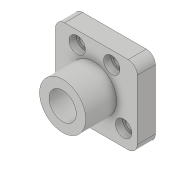
# Autodesk Inventor part: Mount_DMD_KM100
Saved by Autodesk Inventor 2019 (Build 230136000, 136)
## iProperties
Created: 2021-07-26
Part Number: Mount_DMD_KM100
Material: Generic
Document SubType Name: Modeling
Designer: wanghaoran
Density: 1 g/cm^3
Appearance: Default
Author: wanghaoran
Autodesk Inventor part; units mm, degrees
ref_plane "YZ Plane" through (0, 0, 0) normal (1, 0, 0) x (0, 1, 0)
ref_plane "XZ Plane" through (0, 0, 0) normal (0, 1, 0) x (-1, 0, 0)
ref_plane "XY Plane" through (0, 0, 0) normal (0, 0, 1) x (1, 0, 0)
sketch "Sketch1" plane through (0, 0, 0) normal (0, 0, 1) x (1, 0, 0)
  circle A0 centre (19, 0) radius 4.65 projected
  circle A1 centre (-6.5, -27) radius 4.65 projected
  circle A2 centre (0, 0) radius 4.65 projected
  circle A3 centre (25.5, -27) radius 4.65 projected
  arc A4 (28.02, -35.95) -> (33.02, -30.95) centre (28.02, -30.95) ccw projected
  line L0 (33.02, 2.05) -> (33.02, -30.95) projected
  arc A5 (33.02, 2.05) -> (28.02, 7.05) centre (28.02, 2.05) ccw projected
  line L1 (-6.98, 7.05) -> (28.02, 7.05) projected
  arc A6 (-6.98, 7.05) -> (-11.98, 2.05) centre (-6.98, 2.05) ccw projected
  line L2 (-11.98, -30.95) -> (-11.98, 2.05) projected
  arc A7 (-11.98, -30.95) -> (-6.98, -35.95) centre (-6.98, -30.95) ccw projected
  line L3 (28.02, -35.95) -> (-6.98, -35.95) projected
  arc A8 (20.169, -15.05) -> (19.169, -16.05) centre (20.169, -16.05) ccw projected
  line L4 (20.169, -15.05) -> (21.169, -15.05) projected
  line L5 (21.169, -15.05) -> (21.169, -17.95) projected
  line L6 (21.169, -17.95) -> (20.169, -17.95) projected
  arc A9 (19.169, -16.95) -> (20.169, -17.95) centre (20.169, -16.95) ccw projected
  line L7 (19.169, -16.95) -> (19.169, -22.1) projected
  line L8 (19.169, -22.1) -> (-2.331, -22.1) projected
  line L9 (-2.331, -22.1) -> (-2.331, -10.9) projected
  line L10 (-2.331, -10.9) -> (19.169, -10.9) projected
  line L11 (19.169, -10.9) -> (19.169, -16.05) projected
  circle A10 centre (-6.48, -12.9) radius 2 projected
  circle A11 centre (-3.844, -16.512) radius 0.75 projected
  circle A12 centre (23.72, -20.1) radius 2 projected
  line L12 (19.169, -16.05) -> (19.169, -16.95)
  circle A13 centre (25.5, -27) radius 3
  circle A14 centre (-6.5, -27) radius 3
  circle A15 centre (0, 0) radius 3
  circle A16 centre (19, 0) radius 3
  circle A17 centre (19, 0) radius 5
  dimension "d8" = 10
  dimension "d13" = 6
  dimension "d14" = 6
  dimension "d15" = 6
  dimension "d16" = 6
  constraints: 5 centre point, 2 end point, 1 coincident, 1 collinear, 1 tangent
  measures "d8" diameter of A17
  measures "d13" diameter of A16
  measures "d14" diameter of A15
  measures "d15" diameter of A14
  measures "d16" diameter of A13
extrude "Extrusion1" add sketch "Sketch1" along normal blind 10 contours A0 | A1 | A2 | A3 | L3 A7 L2 A6 L1 A5 L0 A4 | L4 L5 L6 A9 L12 A8 | L12 L7 L8 L9 L10 L11 | A10 | A11 | A12 | A17
sketch "Sketch3" plane through (0, 0, 10) normal (0, 0, 1) x (1, 0, 0)
  line L0 (32.9618, -36.0107) -> (-11.98, 7.05)
  line L1 (-11.98, -35.95) -> (33.02, 7.05)
  circle A0 centre (8.9711, -16.071) radius 12.7
  circle A1 centre (-6.5, -27) radius 3 projected
  circle A2 centre (19, 0) radius 3 projected
  point P0 (0, 0)
  dimension "d2" = 25.4
  dimension "d17" = 2.2
  constraints: 4 end point, 1 centre point
  measures "d2" diameter of A0
  measures "d17" distance from line of L0 A0.centre
extrude "Extrusion2" add sketch "Sketch3" along normal blind 17 contours A0 L1 L0 | L0 L1 A0 | L1 A0 L0 | L0 A0 L1
sketch "Sketch4" plane through (8.9711, -16.071, 27) normal (0, 0, 1) x (1, 0, 0)
  circle A0 centre (0, 0) radius 12.7 projected
  circle A1 centre (0, 0) radius 7.5
  point P0 (-8.9711, 16.071)
  dimension "d5" = 15
  constraints: 1 centre point, 1 coincident
  measures "d5" diameter of A1
extrude "Extrusion3" cut sketch "Sketch4" against normal through all contours A1
sketch "Sketch5" plane through (0, 0, 10) normal (0, 0, 1) x (1, 0, 0)
  circle A0 centre (19, 0) radius 3 projected
  circle A1 centre (19, 0) radius 4.5
  circle A2 centre (0, 0) radius 4.5
  circle A3 centre (25.5, -27) radius 3 projected
  circle A4 centre (25.5, -27) radius 4.5
  circle A5 centre (-6.5, -27) radius 3 projected
  circle A6 centre (-6.5, -27) radius 4.5
  dimension "d9" = 9
  dimension "d10" = 9
  dimension "d18" = 9
  dimension "d19" = 9
  constraints: 4 centre point, 4 coincident
  measures "d9" diameter of A1
  measures "d10" diameter of A2
  measures "d18" diameter of A4
  measures "d19" diameter of A6
extrude "Extrusion4" cut sketch "Sketch5" against normal blind 4
body "Solid1"
